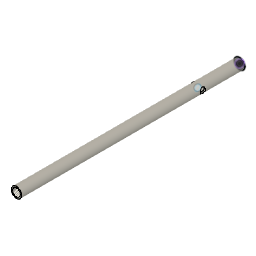
push rod v2 (Autodesk Fusion 360 design; units mm, degrees)
Autodesk Fusion 360 part; units mm, degrees
sketch "Sketch1" plane through (0, 0, 0) normal (0, 0, 1) x (1, 0, 0)
  circle A0 centre (0, 0) radius 4.7625
  circle A1 centre (0, 0) radius 3.5179
  dimension "d1" = 9.525
  dimension "d2" = 7.0358
  constraint coincident A0.centre A1.centre
  measures "d1" diameter of A0
  measures "d2" diameter of A1
extrude "Extrude1" add sketch "Sketch1" along normal blind 203.2
sketch "Sketch2" plane through (0, 0, 0) normal (1, 0, 0) x (0, 0, -1)
  circle A0 centre (-38.1, 0) radius 2.4765
  dimension "d5" = 4.953
  dimension "d6" = 38.1
  measures "d5" diameter of A0
  measures "d6" distance of A0.centre origin
extrude "Extrude2" cut sketch "Sketch2" along normal through all and the other way through all
thread "Thread1" "ANSI Unified Screw Threads 0.3125 5/16-24 UNF 3B" major diameter 7.9375 minor diameter 6.8885 pitch 1.0583 angle 60 resizes the face on face at (3.5126, -0.1939, 94.7614) from (0, 0, 165.1) to (0, 0, 203.2)
